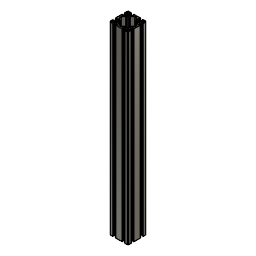
LDO_153030 (Autodesk Fusion 360 design; units mm, degrees)
Autodesk Fusion 360 part; units mm, degrees
sketch "Sketch1" plane through (0, 0, 0) normal (0, 0, 1) x (1, 0, 0)
  line L0 (-15, -15) -> (15, -15)
  line L1 (15, -15) -> (15, 15)
  line L2 (15, 15) -> (-15, 15)
  line L3 (-15, 15) -> (-15, -15)
  line L4 (-15, -15) -> (15, 15) construction
  line L5 (15, -15) -> (-15, 15) construction
  line L6 (-15, 9) -> (-14, 9)
  line L7 (-14, 9) -> (-14, 10.4)
  line L8 (-14, 10.4) -> (-11, 10.4)
  line L9 (-11, 10.4) -> (-9.8, 9.2)
  line L10 (-9.8, 9.2) -> (-9.8, 5.8)
  line L11 (-9.8, 5.8) -> (-11, 4.6)
  line L12 (-11, 4.6) -> (-14, 4.6)
  line L13 (-14, 4.6) -> (-14, 6)
  line L14 (-14, 6) -> (-15, 6)
  line L15 (-9.8, 7.5) -> (-15, 7.5) construction
  circle A0 centre (-7.5, 7.5) radius 1.25
  circle A1 centre (-12.65, 12.65) radius 1.5
  line L16 (-12.5, 1.4029) -> (-12.5, 0)
  line L17 (-12.5, 1.4029) -> (-8.7029, 5.2)
  line L18 (-9.2, 5.2) -> (-5.8, 5.2)
  arc A2 (-7.5, 5.2) -> (-7.5, 6.25) centre (-7.5, 5.725) ccw
  line L19 (-9, 15) -> (-9, 14)
  line L20 (-9, 14) -> (-10.4, 14)
  line L21 (-10.4, 14) -> (-10.4, 11)
  line L22 (-10.4, 11) -> (-9.2, 9.8)
  line L23 (-9.2, 9.8) -> (-5.8, 9.8)
  line L24 (-5.8, 9.8) -> (-4.6, 11)
  line L25 (-4.6, 14) -> (-6, 14)
  line L26 (-6, 14) -> (-6, 15)
  line L27 (-4.6, 11) -> (-4.6, 14)
  line L28 (-1.4029, 12.5) -> (0, 12.5)
  line L29 (-1.4029, 12.5) -> (-5.2, 8.7029)
  line L30 (-5.2, 9.2) -> (-5.2, 5.8)
  arc A3 (-6.25, 7.5) -> (-5.2, 7.5) centre (-5.725, 7.5) ccw
  line L31 (-5.2, -9.2) -> (-5.2, -5.8)
  line L32 (-1.4029, -12.5) -> (0, -12.5)
  line L33 (-1.4029, -12.5) -> (-5.2, -8.7029)
  arc A4 (-5.2, -7.5) -> (-6.25, -7.5) centre (-5.725, -7.5) ccw
  circle A5 centre (-7.5, -7.5) radius 1.25
  arc A6 (-7.5, -6.25) -> (-7.5, -5.2) centre (-7.5, -5.725) ccw
  line L34 (-12.5, -1.4029) -> (-12.5, 0)
  line L35 (-12.5, -1.4029) -> (-8.7029, -5.2)
  line L36 (-15, -9) -> (-14, -9)
  line L37 (-14, -9) -> (-14, -10.4)
  line L38 (-14, -10.4) -> (-11, -10.4)
  line L39 (-11, -10.4) -> (-9.8, -9.2)
  line L40 (-9.8, -9.2) -> (-9.8, -5.8)
  line L41 (-11, -4.6) -> (-14, -4.6)
  line L42 (-14, -4.6) -> (-14, -6)
  line L43 (-14, -6) -> (-15, -6)
  line L44 (-9.8, -5.8) -> (-11, -4.6)
  line L45 (-9.2, -5.2) -> (-5.8, -5.2)
  line L46 (-9, -15) -> (-9, -14)
  line L47 (-9, -14) -> (-10.4, -14)
  line L48 (-10.4, -14) -> (-10.4, -11)
  line L49 (-9.2, -9.8) -> (-5.8, -9.8)
  line L50 (-5.8, -9.8) -> (-4.6, -11)
  line L51 (-4.6, -11) -> (-4.6, -14)
  line L52 (-4.6, -14) -> (-6, -14)
  line L53 (-6, -14) -> (-6, -15)
  line L54 (-10.4, -11) -> (-9.2, -9.8)
  circle A7 centre (-12.65, -12.65) radius 1.5
  line L55 (9.2, -5.2) -> (5.8, -5.2)
  line L56 (12.5, -1.4029) -> (12.5, 0)
  line L57 (12.5, -1.4029) -> (8.7029, -5.2)
  arc A8 (7.5, -5.2) -> (7.5, -6.25) centre (7.5, -5.725) ccw
  circle A9 centre (7.5, -7.5) radius 1.25
  arc A10 (6.25, -7.5) -> (5.2, -7.5) centre (5.725, -7.5) ccw
  line L58 (1.4029, -12.5) -> (0, -12.5)
  line L59 (1.4029, -12.5) -> (5.2, -8.7029)
  line L60 (9, -15) -> (9, -14)
  line L61 (9, -14) -> (10.4, -14)
  line L62 (10.4, -14) -> (10.4, -11)
  line L63 (10.4, -11) -> (9.2, -9.8)
  line L64 (9.2, -9.8) -> (5.8, -9.8)
  line L65 (4.6, -11) -> (4.6, -14)
  line L66 (4.6, -14) -> (6, -14)
  line L67 (6, -14) -> (6, -15)
  line L68 (5.8, -9.8) -> (4.6, -11)
  line L69 (5.2, -9.2) -> (5.2, -5.8)
  line L70 (15, -9) -> (14, -9)
  line L71 (14, -9) -> (14, -10.4)
  line L72 (14, -10.4) -> (11, -10.4)
  line L73 (9.8, -9.2) -> (9.8, -5.8)
  line L74 (9.8, -5.8) -> (11, -4.6)
  line L75 (11, -4.6) -> (14, -4.6)
  line L76 (14, -4.6) -> (14, -6)
  line L77 (14, -6) -> (15, -6)
  line L78 (11, -10.4) -> (9.8, -9.2)
  circle A11 centre (12.65, -12.65) radius 1.5
  line L79 (5.2, 9.2) -> (5.2, 5.8)
  line L80 (1.4029, 12.5) -> (0, 12.5)
  line L81 (1.4029, 12.5) -> (5.2, 8.7029)
  arc A12 (5.2, 7.5) -> (6.25, 7.5) centre (5.725, 7.5) ccw
  circle A13 centre (7.5, 7.5) radius 1.25
  arc A14 (7.5, 6.25) -> (7.5, 5.2) centre (7.5, 5.725) ccw
  line L82 (12.5, 1.4029) -> (12.5, 0)
  line L83 (12.5, 1.4029) -> (8.7029, 5.2)
  line L84 (15, 9) -> (14, 9)
  line L85 (14, 9) -> (14, 10.4)
  line L86 (14, 10.4) -> (11, 10.4)
  line L87 (11, 10.4) -> (9.8, 9.2)
  line L88 (9.8, 9.2) -> (9.8, 5.8)
  line L89 (11, 4.6) -> (14, 4.6)
  line L90 (14, 4.6) -> (14, 6)
  line L91 (14, 6) -> (15, 6)
  line L92 (9.8, 5.8) -> (11, 4.6)
  line L93 (9.2, 5.2) -> (5.8, 5.2)
  line L94 (9, 15) -> (9, 14)
  line L95 (9, 14) -> (10.4, 14)
  line L96 (10.4, 14) -> (10.4, 11)
  line L97 (9.2, 9.8) -> (5.8, 9.8)
  line L98 (5.8, 9.8) -> (4.6, 11)
  line L99 (4.6, 11) -> (4.6, 14)
  line L100 (4.6, 14) -> (6, 14)
  line L101 (6, 14) -> (6, 15)
  line L102 (10.4, 11) -> (9.2, 9.8)
  circle A15 centre (12.65, 12.65) radius 1.5
  dimension "d1" = 30
  dimension "d2" = 3
  dimension "d3" = 5.2
  dimension "d4" = 5.8
  dimension "d5" = 7.5
  dimension "d6" = 1
  dimension "d7" = 135
  dimension "d8" = 3
  dimension "d9" = 7.5
  dimension "d10" = 2.5
  dimension "d11" = 3
  dimension "d12" = 2.35
  dimension "d13" = 2.5
  dimension "d14" = 1.2
  dimension "d16" = 90
  dimension "d18" = 360
  constraint horizontal L0
  constraint perpendicular L0 L1
  constraint parallel L0 L2
  constraint parallel L1 L3
  constraint coincident L4 origin
  constraint coincident L5 origin
  constraint equal L0 L3
  constraint coincident L3 L6.start
  constraint perpendicular L3 L6
  constraint perpendicular L6 L7
  constraint perpendicular L7 L8
  constraint perpendicular L6 L10
  constraint perpendicular L10 L12
  constraint perpendicular L12 L13
  constraint coincident L3 L14.end
  constraint perpendicular L3 L14
  constraint equal L6 L14
  constraint equal L9 L11
  constraint midpoint L10 L15.start
  constraint coincident L3 L15.end
  constraint perpendicular L3 L15
  constraint symmetric L6 L14 L15
  constraint symmetric L8 L12 L15
  constraint coincident L5 A0.centre
  constraint coincident L5 A1.centre
  constraint parallel L3 L16
  constraint parallel L11 L17
  constraint coincident L17.end L18
  constraint tangent L18 A2
  constraint coincident L18 A2.start
  constraint coincident A0 A2.end
  constraint tangent A0 A2
  constraint vertical A0.centre A2.centre
  constraint symmetric L5 L6.start L19.start
  constraint symmetric L5 L6.end L19.end
  constraint symmetric L5 L7.end L20.end
  constraint symmetric L5 L8.end L21.end
  constraint symmetric L5 L9.end L22.end
  constraint symmetric L5 L10.end L23.end
  constraint symmetric L5 L11.end L24.end
  constraint symmetric L5 L12.end L25.start
  constraint symmetric L5 L13.end L25.end
  constraint symmetric L5 L14.end L26.end
  constraint symmetric L5 L16.start L28.start
  constraint symmetric L5 L16.end L28.end
  constraint symmetric L5 L17.end L29.end
  constraint symmetric L5 L18.start L30.start
  constraint symmetric L5 L18.end L30.end
  constraint symmetric L5 A2.end A3.start
  constraint symmetric L5 A2.start A3.end
  constraint symmetric L5 A2 A3
  constraint horizontal origin L16.end
  measures "d1" distance of L0.start L0.end
  measures "d2" distance of L6 L14
  measures "d3" distance of L3 L10
  measures "d4" distance of L8 L12
  measures "d5" distance of L2 L15
  measures "d6" distance of L3 L7
  measures "d7" angle of L9 L10
  measures "d8" distance of L7 L8.end
  measures "d9" distance of L3 A0.centre
  measures "d10" diameter of A0
  measures "d11" diameter of A1
  measures "d12" distance of L3 A1.centre
  measures "d13" distance of L3 L16
  measures "d14" distance of L11 L17
extrude "Extrude1" add sketch "Sketch1" along normal blind 300 contours L0 L1 L2 L3 L6 L7 L8 L9 L10 L11 L12 L13 L14 L19 L20 L21 L22 L23 L24 L25 L26 L27 L36 L37 L38 L39 L40 L41 L42 L43 L44 L46 L47 L48 L49 L50 L51 L52 L53 L54 L60 L61 L62 L63 L64 L65 L66 L67 L68 L70 L71 L72 L73 L74 L75 L76 L77 L78 L84 L85 L86 L87 L88 L89 L90 L91 L92 L94 L95 L96 L97 L98 L99 L100 L101 L102
fillet "Fillet1" radius 0.4 32 edges at (-14, 6, 150) (-15, 6, 150) (-15, 9, 150) (-14, 9, 150) (-9, 14, 150) (-9, 15, 150) (-6, 14, 150) (-6, 15, 150) (-15, -6, 150) (-14, -6, 150) (-14, -9, 150) (-15, -9, 150) (-9, -15, 150) (-9, -14, 150) (-6, -14, 150) (-6, -15, 150) (6, -15, 150) (6, -14, 150) (9, -14, 150) (9, -15, 150) (15, -9, 150) (14, -9, 150) (15, -6, 150) (14, -6, 150) (15, 6, 150) (14, 6, 150) (15, 9, 150) (14, 9, 150) (9, 14, 150) (9, 15, 150) (6, 14, 150) (6, 15, 150)
fillet "Fillet1" radius 1 4 edges at (-15, 15, 150) (15, 15, 150) (15, -15, 150) (-15, -15, 150)
equation "d12 = 0.85 mm + 1.5 mm"
equation "Extrusion_Length = 300 mm"
equation "d20 = Extrusion_Length"
